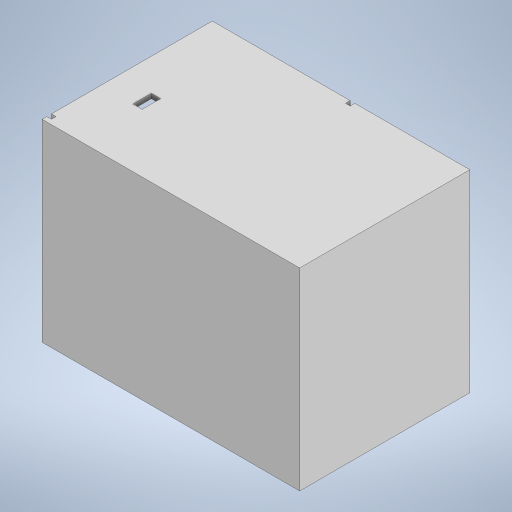
# Autodesk Inventor part: lid
Saved by Autodesk Inventor 2024 (Build 280153000, 153)
## iProperties
Created: 2024-04-17
Part Number: lid
Material: Generic
Document SubType Name: Modeling
Designer: 22546723
Density: 1 g/cm^3
Appearance: Default
Author: 22546723
## iProperties of the stored document lid_3DPrint.ipt
Created: 2024-04-17
Part Number: lid_3DPrint
Material: Generic
Document SubType Name: Modeling
Designer: 22546723
Density: 1 g/cm^3
Appearance: Default
Author: 22546723
Autodesk Inventor part; units mm, degrees
ref_plane "YZ Plane" through (0, 0, 0) normal (1, 0, 0) x (0, 1, 0)
ref_plane "XZ Plane" through (0, 0, 0) normal (0, 1, 0) x (-1, 0, 0)
ref_plane "XY Plane" through (0, 0, 0) normal (0, 0, 1) x (1, 0, 0)
sketch "Sketch1" plane through (0, 0, 0) normal (0, 1, 0) x (-1, 0, 0)
  line L0 (58, 35) -> (-50, 35)
  line L1 (-50, 35) -> (-50, -35)
  line L2 (-50, -35) -> (58, -35)
  line L3 (58, -35) -> (58, 35)
  point P0 (0, 0)
  dimension "d1" = 70
  dimension "d36" = 50
  dimension "d37" = 58
  dimension "d38" = 35
  constraints: 8 end point, 2 parallel, 1 horizontal, 1 perpendicular
  measures "d1" distance between parallel lines of L0 L2
  measures "d36" distance from line of L1 point (0, 0)
  measures "d37" distance from line of L3 point (0, 0)
  measures "d38" distance from line of point (0, 0) L2
extrude "Extrusion1" add sketch "Sketch1" against normal blind 2
sketch "Sketch2" plane through (0, 0, 0) normal (0, 1, 0) x (-1, 0, 0)
  line L0 (-50, 35) -> (58, 35) projected
  line L1 (58, 35) -> (-50, 35)
  line L2 (-50, 35) -> (-50, 37)
  line L3 (-50, 37) -> (58, 37)
  line L4 (58, 37) -> (58, 35)
  point P0 (0, 0)
  dimension "d4" = 2
  constraints: 8 end point, 2 parallel, 1 horizontal, 1 perpendicular, 1 point on line
  measures "d4" distance between parallel lines of L0 L3
extrude "Extrusion2" add sketch "Sketch2" against normal blind 84
sketch "Sketch3" plane through (0, 0, 0) normal (0, 1, 0) x (-1, 0, 0)
  line L0 (58, -35) -> (-50, -35) projected
  line L1 (-50, -35) -> (-52, -35)
  line L2 (-52, -35) -> (-52, 37)
  line L3 (-52, 37) -> (-50, 37)
  line L4 (-50, 37) -> (-50, -35)
  point P0 (0, 0)
  dimension "d7" = 2
  constraints: 8 end point, 2 parallel, 1 horizontal, 1 perpendicular
  measures "d7" distance of L3.end L2.end
extrude "Extrusion3" add sketch "Sketch3" against normal blind 84
sketch "Sketch4" plane through (0, 0, 0) normal (0, 1, 0) x (-1, 0, 0)
  line L0 (-50, -35) -> (-52, -35) projected
  line L1 (-52, -35) -> (-2, -35)
  line L2 (-2, -35) -> (-2, -37)
  line L3 (-2, -37) -> (-52, -37)
  line L4 (-52, -37) -> (-52, -35)
  point P0 (0, 0)
  dimension "d10" = 50
  dimension "d11" = 2
  constraints: 8 end point, 2 parallel, 1 horizontal, 1 perpendicular
  measures "d10" distance of L2.end L3.end
  measures "d11" distance between parallel lines of L1 L3
extrude "Extrusion4" add sketch "Sketch4" against normal blind 71
sketch "Sketch5" plane through (52, 0, -37) normal (0, 0, -1) x (-1, 0, 0)
  line L0 (50, -2) -> (50, -71) projected
  line L1 (50, -71) -> (46, -71)
  line L2 (46, -71) -> (46, -59)
  line L3 (46, -59) -> (50, -59)
  line L4 (50, -59) -> (50, -71)
  point P0 (52, 0)
  dimension "d14" = 4
  dimension "d15" = 12
  constraints: 8 end point, 2 parallel, 1 horizontal, 1 perpendicular
  measures "d14" distance of L2.end L3.end
  measures "d15" distance between parallel lines of L1 L3
extrude "Extrusion5" cut sketch "Sketch5" against normal blind 3
sketch "Sketch6" plane through (0, 0, 0) normal (0, 1, 0) x (-1, 0, 0)
  line L0 (58, -35) -> (58, 37) projected
  line L1 (58, 37) -> (60, 37)
  line L2 (60, 37) -> (60, -37)
  line L3 (-2, -37) -> (-2, -35) projected
  line L4 (60, -37) -> (-2, -37)
  line L5 (58, -35) -> (-2, -35) projected
  line L6 (-2, -37) -> (-2, -35)
  point P0 (0, 0)
  dimension "d18" = 2
  constraints: 8 end point, 2 horizontal, 1 parallel, 1 perpendicular
  measures "d18" distance of L0.end L1.end
extrude "Extrusion6" add sketch "Sketch6" against normal blind 2
sketch "Sketch7" plane through (0, -2, 0) normal (0, -1, 0) x (1, 0, 0)
  line L0 (2, -35) -> (2, -37) projected
  line L1 (2, -37) -> (0, -37)
  line L2 (0, -37) -> (0, -35)
  line L3 (0, -35) -> (2, -35)
  line L4 (2, -35) -> (2, -37)
  line L5 (2, -37) -> (2, -35) projected
  point P0 (0, 0)
  point P1 (1, -37)
  point P2 (1, -35)
  point P3 (2, -36)
  point P4 (0, -36)
  dimension "d21" = 2
  dimension "d22" = 2
  constraints: 8 end point, 4 midpoint, 2 parallel, 1 horizontal, 1 perpendicular
  measures "d21" distance of point (1, -37) point (1, -35)
  measures "d22" distance of point (2, -36) point (0, -36)
sketch "Sketch8" plane through (0, -2, 0) normal (0, -1, 0) x (1, 0, 0)
  line L0 (50, 35) -> (-58, 35) projected
  line L1 (-60, 37) -> (-60, -37) projected
  line L2 (-58, 35) -> (-60, 35)
  line L3 (-60, 35) -> (-60, 37)
  line L4 (-60, 37) -> (-58, 37)
  line L5 (-58, 37) -> (-58, 35)
  point P0 (0, 0)
  constraints: 8 end point, 2 parallel, 1 horizontal, 1 perpendicular
extrude "Extrusion7" add sketch "Sketch8" along normal blind 82
sketch "Sketch9" plane through (0, -2, 0) normal (0, -1, 0) x (1, 0, 0)
  line L0 (-60, 37) -> (-60, 35) projected
  line L1 (-60, 35) -> (-58, 35)
  line L2 (-58, 35) -> (-58, 33)
  line L3 (-58, 33) -> (-60, 33)
  line L4 (-60, 33) -> (-60, 35)
  point P0 (0, 0)
  dimension "d25" = 2
  dimension "d26" = 2
  constraints: 8 end point, 2 parallel, 1 horizontal, 1 perpendicular
  measures "d25" distance of L2.end L3.end
  measures "d26" distance between parallel lines of L1 L3
extrude "Extrusion8" cut sketch "Sketch9" against normal blind 2
extrude "Extrusion9" cut sketch "Sketch7" against normal blind 2
sketch "Sketch10" plane through (0, -71, 0) normal (0, -1, 0) x (1, 0, 0)
  line L0 (52, 37) -> (52, -37) projected
  line L1 (2, -35) -> (50, -35) projected
  line L2 (52, -37) -> (50, -37)
  line L3 (50, -37) -> (50, -35)
  line L4 (50, -35) -> (52, -35)
  line L5 (52, -35) -> (52, -37)
  point P0 (0, 0)
  constraints: 8 end point, 2 parallel, 1 horizontal, 1 perpendicular
extrude "Extrusion10" add sketch "Sketch10" along normal blind 13
sketch "Sketch11" plane through (0, -71, 0) normal (0, -1, 0) x (1, 0, 0)
  line L0 (50, 35) -> (50, -37) projected
  line L1 (50, -35) -> (6, -35) projected
  line L2 (50, -37) -> (48, -37)
  line L3 (48, -37) -> (48, -35)
  line L4 (48, -35) -> (50, -35)
  line L5 (50, -35) -> (50, -37)
  point P0 (0, 0)
  dimension "d33" = 2
  constraints: 8 end point, 2 parallel, 1 horizontal, 1 perpendicular, 1 point on line
  measures "d33" distance of L3.end L4.end
extrude "Extrusion11" cut sketch "Sketch11" against normal blind 2
sketch "Sketch12" plane through (0, 0, 0) normal (0, 1, 0) x (1, 0, 0)
  line L0 (-42, -3.5) -> (-46, -3.5)
  line L1 (-46, -3.5) -> (-46, -11.5)
  line L2 (-46, -11.5) -> (-42, -11.5)
  line L3 (-42, -11.5) -> (-42, -3.5)
  line L4 (-42, -3.5) -> (-46, -11.5) construction
  line L5 (-46, -3.5) -> (-42, -11.5) construction
  line L6 (0, 37) -> (-60, 37) projected
  line L7 (-60, 37) -> (-60, -33) projected
  point P0 (0, 0)
  point P1 (-44, -7.5)
  dimension "d39" = 44.5
  dimension "d41" = 4
  dimension "d42" = 8
  dimension "d43" = 14
  constraints: 12 end point, 2 midpoint, 2 parallel, 1 horizontal, 1 perpendicular
  measures "d39" distance from line of L6 point (-44, -7.5)
  measures "d41" distance between parallel lines of L1 L3
  measures "d42" distance between parallel lines of L0 L2
  measures "d43" distance between parallel lines of L7 L1
extrude "Extrusion12" cut sketch "Sketch12" against normal blind 10
body "Solid1"
